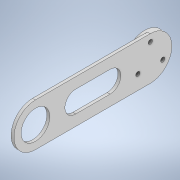
# Autodesk Inventor part: psmall
Saved by Autodesk Inventor 2022 (Build 260153000, 153)
## iProperties
Created: 2022-03-17
Part Number: psmall
Material: Generic
Document SubType Name: Modeling
Designer: br4ch
Density: 1 g/cm^3
Appearance: Default
Author: br4ch
Autodesk Inventor part; units mm, degrees
ref_plane "YZ Plane" through (0, 0, 0) normal (1, 0, 0) x (0, 1, 0)
ref_plane "XZ Plane" through (0, 0, 0) normal (0, 1, 0) x (-1, 0, 0)
ref_plane "XY Plane" through (0, 0, 0) normal (0, 0, 1) x (1, 0, 0)
sketch "Sketch1" plane through (0, 0, 0) normal (1, 0, 0) x (0, 1, 0)
  line L0 (5.01, 17.9997) -> (5.01, -62.0003) construction
  line L1 (-9.99, 17.9997) -> (-9.99, -62.0003)
  line L2 (20.01, -62.0003) -> (20.01, 17.9997)
  arc A0 (20.01, 17.9997) -> (-9.99, 17.9997) centre (5.01, 17.9997) ccw
  arc A1 (-9.99, -62.0003) -> (20.01, -62.0003) centre (5.01, -62.0003) ccw
  circle A2 centre (5.01, 17.9997) radius 10
  line L3 (5.01, -10.0003) -> (5.01, -34.0003) construction
  line L4 (-2.49, -10.0003) -> (-2.49, -34.0003)
  line L5 (12.51, -34.0003) -> (12.51, -10.0003)
  arc A3 (12.51, -10.0003) -> (-2.49, -10.0003) centre (5.01, -10.0003) ccw
  arc A4 (-2.49, -34.0003) -> (12.51, -34.0003) centre (5.01, -34.0003) ccw
  line L6 (-8.9091, -22.0003) -> (18.0909, -22.0003) construction
  circle A5 centre (5.01, -62.0003) radius 10 construction
  circle A6 centre (15.01, -62.0003) radius 1.5
  circle A7 centre (0.01, -53.34) radius 1.5
  circle A8 centre (0.01, -70.6605) radius 1.5
  circle A9 centre (5.01, -62.0003) radius 15
  point P0 (0, 0)
  point P1 (5.01, -22.0003)
  point P2 (-9.99, -62.0003)
  dimension "d0" = 30
  dimension "d1" = 80
  dimension "d2" = 20
  dimension "d5" = 15
  dimension "d6" = 3
  dimension "d9" = 360
  dimension "d13" = 24
  constraints: 18 end point, 8 centre point, 8 point on circle, 8 tangent, 2 coincident, 2 midpoint, 2 parallel, 2 point on line, 1 horizontal alignment, 1 perpendicular, 1 symmetric about line, 1 vertical, 13 other
  measures "d0" diameter of A1
  measures "d1" distance of L2.start L2.end
  measures "d2" diameter of A2
  measures "d5" diameter of A4
  measures "d6" diameter of A6
  measures "d13" distance of L4.start L4.end
extrude "Extrusion1" add sketch "Sketch1" along normal blind 2
extrude "Extrusion2" add sketch "Sketch1" against normal blind 2 contours A9 A1
body "Solid1"
